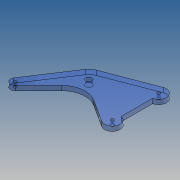
# Autodesk Inventor part: Protector
Saved by Autodesk Inventor 2017 (Build 210142000, 142)
## iProperties
Part Number: Protector
Material: Genérico
Document SubType Name: Modeling
Designer: Leo
Density: 1 g/cm^3
Appearance: Claro - Azul
Author: Leo
Autodesk Inventor part; units mm, degrees
ref_plane "YZ Plane" through (0, 0, 0) normal (1, 0, 0) x (0, 1, 0)
ref_plane "XZ Plane" through (0, 0, 0) normal (0, 1, 0) x (-1, 0, 0)
ref_plane "XY Plane" through (0, 0, 0) normal (0, 0, 1) x (1, 0, 0)
sketch "Boceto1" plane through (0, 0, 0) normal (0, 0, 1) x (1, 0, 0)
  circle A0 centre (22.1541, -50) radius 2 projected
  circle A1 centre (127.9669, -30) radius 2 projected
  circle A2 centre (127.9669, 30) radius 2 projected
  line L0 (17.1394, -46.7056) -> (53.7548, 9.0299)
  line L1 (61.631, 15.3631) -> (124.3983, 39.3415)
  arc A3 (129.9669, 20.202) -> (124.3983, 39.3415) centre (127.9669, 30) ccw
  line L2 (129.9669, 20.202) -> (129.9669, -20.202)
  arc A4 (122.5476, -38.4042) -> (129.9669, -20.202) centre (127.9669, -30) ccw
  line L3 (122.5476, -38.4042) -> (94.108, -20.0654)
  line L4 (56.6587, -24.043) -> (26.3924, -54.247)
  arc A5 (17.1394, -46.7056) -> (26.3924, -54.247) centre (22.1541, -50) ccw
  arc A6 (61.631, 15.3631) -> (53.7548, 9.0299) centre (67.5, 0) ccw
  circle A7 centre (67.5, 0) radius 4 projected
  arc A8 (94.108, -20.0654) -> (56.6587, -24.043) centre (77.85, -45.2781) ccw
  point P0 (0, 0)
  point P1 (73.7799, -6.9571)
  dimension "d0" = 10
  dimension "d1" = 8
  dimension "d4" = 6
  dimension "d5" = 30
  constraints: 10 end point, 10 point on circle, 9 tangent, 5 centre point, 4 concentric, 2 point on line, 1 equal radius
  measures "d0" radius of A3
  measures "d1" distance edge to line of A3 L2
  measures "d4" radius of A5
  measures "d5" radius of A8
extrude "Extrusión1" add sketch "Boceto1" along normal blind 6
